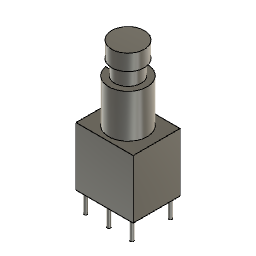
FootSW_DPDT (Autodesk Fusion 360 design; units mm, degrees)
Autodesk Fusion 360 part; units mm, degrees
sketch "スケッチ1" plane through (0, 0, 0) normal (0, 0, 1) x (1, 0, 0)
  line L0 (-8.6, -7.05) -> (8.6, -7.05)
  line L1 (8.6, -7.05) -> (8.6, 7.05)
  line L2 (8.6, 7.05) -> (-8.6, 7.05)
  line L3 (-8.6, 7.05) -> (-8.6, -7.05)
  line L4 (-10.1, 0) -> (-7.1, 0) construction
  line L5 (0, -5.05) -> (0, -9.05) construction
  line L6 (0, 1.75) -> (0, 22.5)
  line L7 (1.75, 0) -> (22.5, 0)
  circle A0 centre (0, 5.75) radius 0.5
  circle A1 centre (-7, 5.75) radius 0.5
  circle A2 centre (7, 5.75) radius 0.5
  circle A3 centre (0, -5.75) radius 0.5
  circle A4 centre (-7, -5.75) radius 0.5
  circle A5 centre (7, -5.75) radius 0.5
  dimension "d1" = 17.2
  dimension "d2" = 14.1
  dimension "d5" = 1
  dimension "d6" = 1.3
  dimension "d9" = 7
  dimension "d10" = -5
  constraint horizontal L0
  constraint vertical L1
  constraint horizontal L2
  constraint vertical L3
  constraint perpendicular L3 L4
  constraint vertical L5
  constraint midpoint L3 L4
  constraint midpoint L0 L5
  constraint collinear L5 L6
  constraint collinear L4 L7
  constraint coincident L6 A0.centre
  constraint symmetric L7 A0 A3
  constraint symmetric L7 A1 A4
  constraint symmetric L7 A2 A5
  measures "d1" distance of L0.start L0.end
  measures "d2" distance of L0.start L2.end
  measures "d5" diameter of A0
  measures "d6" distance of L2 A0.centre
extrude "押し出し1" add sketch "スケッチ1" along normal blind 17.6 contours L0 L1 L2 L3 | L6 A0 | L6 A0 | A1 | A2 | A3 | A4 | A5
extrude "押し出し2" add sketch "スケッチ1" against normal blind 6 contours L6 A0 | L6 A0 | A1 | A2 | A3 | A4 | A5
sketch "スケッチ2" plane through (0, 0, 17.6) normal (0, 0, 1) x (-1, 0, 0)
  line L0 (8.6, -7.05) -> (8.6, 7.05)
  line L1 (8.6, 7.05) -> (-8.6, 7.05)
  line L2 (-8.6, 7.05) -> (-8.6, -7.05)
  line L3 (-8.6, -7.05) -> (8.6, -7.05)
  circle A0 centre (0, 0) radius 5.8
  line L4 (5.8, -1) -> (4.8, -1)
  line L5 (4.8, -1) -> (4.8, 1)
  line L6 (4.8, 1) -> (5.8, 1)
  line L7 (5.8, 1) -> (5.8, -1)
  line L8 (9.063, 0) -> (8.137, 0) construction
  line L9 (6.2854, 0) -> (5.3146, 0) construction
  dimension "d13" = 11.6
  dimension "d14" = 1
  dimension "d15" = 2
  constraint coincident A0.centre origin
  constraint horizontal L4
  constraint vertical L5
  constraint horizontal L6
  constraint vertical L7
  constraint perpendicular L7 L8
  constraint horizontal L9
  constraint midpoint L0 L8
  constraint midpoint L7 L9
  constraint collinear L8 L9
  constraint tangent A0 L7
  measures "d13" diameter of A0
  measures "d14" distance of L4.start L4.end
  measures "d15" distance of L4.start L6.end
extrude "押し出し3" add sketch "スケッチ2" along normal blind 13 contours A0 L4 L5 L6 picked at (1.2667, 0)
sketch "スケッチ3" plane through (0, 0, 30.6) normal (0, 0, 1) x (-1, 0, 0)
  line L0 (4.8, 1) -> (5.7131, 1)
  arc A0 (5.7131, 1) -> (5.7131, -1) centre (0, 0) ccw
  line L1 (5.7131, -1) -> (4.8, -1)
  line L2 (4.8, -1) -> (4.8, 1)
  circle A1 centre (0, 0) radius 4
  dimension "d18" = 8
  constraint coincident A0.centre A1.centre
  measures "d18" diameter of A1
extrude "押し出し4" add sketch "スケッチ3" along normal blind 4.5 contours A1
sketch "スケッチ4" plane through (0, 0, 35.1) normal (0, 0, 1) x (-1, 0, 0)
  circle A0 centre (0, 0) radius 4
  circle A1 centre (0, 0) radius 4.9
  dimension "d21" = 9.8
  constraint concentric A0 A1
  measures "d21" diameter of A1
extrude "押し出し5" add sketch "スケッチ4" along normal blind 4.8 contours A0 | A1
